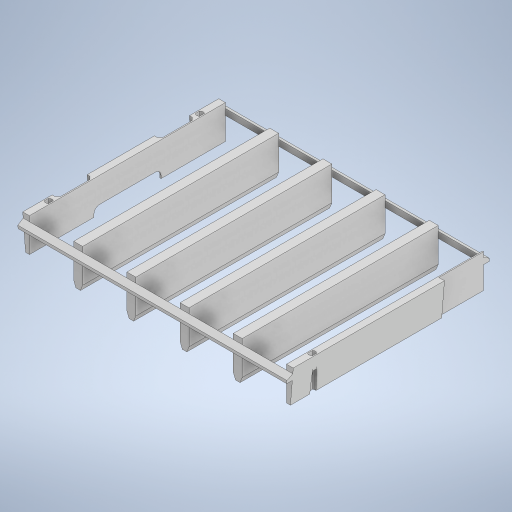
# Autodesk Inventor part: Brackets
Saved by Autodesk Inventor 2023 (Build 270158000, 158)
## iProperties
Created: 2024-03-26
Part Number: Brackets
Material: Generic
Document SubType Name: Modeling
Designer: noname
Density: 1 g/cm^3
Appearance: Default
Author: noname
Autodesk Inventor part; units mm, degrees
ref_plane "YZ Plane" through (0, 0, 0) normal (1, 0, 0) x (0, 1, 0)
ref_plane "XZ Plane" through (0, 0, 0) normal (0, 1, 0) x (-1, 0, 0)
ref_plane "XY Plane" through (0, 0, 0) normal (0, 0, 1) x (1, 0, 0)
sketch "Sketch1" plane through (0, 0, 0) normal (0, 1, 0) x (-1, 0, 0)
  line L0 (0, 0) -> (-96.6, 0) construction
  line L1 (-96.6, 0) -> (-96.6, -70) construction
  line L2 (-96.6, -70) -> (0, -70) construction
  line L3 (0, -70) -> (0, 0) construction
  line L4 (0, 0) -> (-2.4, 0)
  line L5 (-2.4, 0) -> (-2.4, -70)
  line L6 (-2.4, -70) -> (0, -70)
  line L7 (0, -70) -> (0, 0)
  line L8 (-48.3, 0) -> (-48.3, -70)
  line L9 (-96.6, -70) -> (-96.6, 0) construction
  line L10 (-96.6, 0) -> (-94.2, 0)
  line L11 (-94.2, 0) -> (-94.2, -70)
  line L12 (-94.2, -70) -> (-96.6, -70)
  line L13 (-96.6, -70) -> (-96.6, 0)
  line L14 (-18.2, 0) -> (-21.4, 0)
  line L15 (-21.4, 0) -> (-21.4, -70)
  line L16 (-21.4, -70) -> (-18.2, -70)
  line L17 (-18.2, -70) -> (-18.2, 0)
  line L18 (-40.4, 0) -> (-40.4, -70)
  line L19 (-40.4, -70) -> (-37.2, -70)
  line L20 (-37.2, -70) -> (-37.2, 0)
  line L21 (-37.2, 0) -> (-40.4, 0)
  line L22 (-59.4, 0) -> (-59.4, -70)
  line L23 (-59.4, -70) -> (-56.2, -70)
  line L24 (-56.2, -70) -> (-56.2, 0)
  line L25 (-56.2, 0) -> (-59.4, 0)
  line L26 (-78.4, 0) -> (-78.4, -70)
  line L27 (-78.4, -70) -> (-75.2, -70)
  line L28 (-75.2, -70) -> (-75.2, 0)
  line L29 (-75.2, 0) -> (-78.4, 0)
  dimension "d0" = 96.6
  dimension "d1" = 70
  dimension "d2" = 2.4
  dimension "d5" = 19
  dimension "d10" = 19
  dimension "d11" = 3.2
  dimension "d12" = 19
  constraints: 60 end point, 6 parallel, 4 horizontal, 4 symmetric about line, 3 perpendicular, 3 point on line, 2 midpoint, 24 other
  measures "d0" distance between parallel lines of L1 L3
  measures "d1" distance between parallel lines of L0 L2
  measures "d2" distance between parallel lines of L7 L5
  measures "d5" distance of L15.end L18.end
  measures "d10" distance between parallel lines of L5 L15
  measures "d11" distance between parallel lines of L15 L17
  measures "d12" distance between parallel lines of L28 L11
extrude "Extrusion1" add sketch "Sketch1" along normal blind 12
sketch "Sketch2" plane through (0, 0, 0) normal (0, 0, 1) x (1, 0, 0)
  line L0 (18.2, 0) -> (21.4, 0) projected
  line L1 (21.4, 0) -> (21.4, 12) projected
  line L2 (18.2, 12) -> (21.4, 12) projected
  line L3 (18.2, 0) -> (18.2, 12) projected
  line L4 (21.4, 0) -> (18.2, 0) projected
  line L5 (18.2, 0) -> (19, -2)
  line L6 (19, -2) -> (20.6, -2)
  line L7 (20.6, -2) -> (21.4, 0)
  line L8 (18.2, 0) -> (21.4, 0)
  line L9 (37.2, 0) -> (38, -2)
  line L10 (38, -2) -> (39.6, -2)
  line L11 (39.6, -2) -> (40.4, 0)
  line L12 (37.2, 0) -> (40.4, 0)
  line L13 (56.2, 0) -> (57, -2)
  line L14 (57, -2) -> (58.6, -2)
  line L15 (58.6, -2) -> (59.4, 0)
  line L16 (56.2, 0) -> (59.4, 0)
  line L17 (75.2, 0) -> (76, -2)
  line L18 (76, -2) -> (77.6, -2)
  line L19 (77.6, -2) -> (78.4, 0)
  line L20 (75.2, 0) -> (78.4, 0)
  dimension "d17" = 2
  dimension "d18" = 1.6
  dimension "d21" = 19
  constraints: 32 end point, 2 horizontal, 1 equal length, 1 parallel, 24 other
  measures "d17" distance between parallel lines of L0 L6
  measures "d18" distance of L5.end L6.end
  measures "d21" distance of L0.start L9.start
extrude "Extrusion2" add sketch "Sketch2" against normal up to surface (70 mm away) contours L0 L7 L6 L5 | L12 L11 L10 L9 | L16 L15 L14 L13 | L20 L19 L18 L17
sketch "Sketch3" plane through (0, 0, 0) normal (0, 0, 1) x (1, 0, 0)
  line L0 (0, 12) -> (1, 0)
  line L1 (0, 0) -> (0, 12) projected
  line L2 (0, 12) -> (0, 0)
  line L3 (0, 0) -> (1, 0)
  line L4 (40.4, 0) -> (40.4, 12) projected
  line L5 (40.4, 6) -> (56.2, 6) construction
  line L6 (56.2, 0) -> (56.2, 12) projected
  line L7 (48.3, 12) -> (48.3, 0)
  line L8 (96.6, 12) -> (95.6, 0)
  line L9 (96.6, 0) -> (96.6, 12)
  line L10 (96.6, 0) -> (95.6, 0)
  point P0 (48.3, 6)
  dimension "d28" = 1
  constraints: 16 end point, 4 midpoint, 3 symmetric about line, 2 horizontal alignment, 2 vertical, 1 perpendicular
  measures "d28" distance from line of L1 L0.end
extrude "Extrusion3" cut sketch "Sketch3" against normal through all
ref_plane "Work Plane1" through (0, 9, 0) normal (0, 1, 0) x (1, 0, 0)
sketch "Sketch4" plane through (0, 9, 0) normal (0, 1, 0) x (1, 0, 0)
  line L0 (0, 0) -> (2.4, 0) projected
  line L1 (0, 0) -> (96.6, 0)
  line L2 (96.6, 0) -> (96.6, -2)
  line L3 (96.6, -2) -> (0, -2)
  line L4 (0, -2) -> (0, 0)
  line L5 (2.4, 70) -> (0, 70) projected
  line L6 (0, 70) -> (96.6, 70)
  line L7 (96.6, 70) -> (96.6, 72)
  line L8 (96.6, 72) -> (0, 72)
  line L9 (0, 72) -> (0, 70)
  dimension "d32" = 2
  dimension "d36" = 2
  constraints: 16 end point, 4 parallel, 2 horizontal, 2 perpendicular, 2 vertical alignment
  measures "d32" distance between parallel lines of L6 L8
  measures "d36" distance between parallel lines of L3 L1
extrude "Extrusion4" add sketch "Sketch4" against normal blind 1
draft "FaceDraft1" angle 30 pull direction (0, 0, -1) faces at (38.2667, 9, -71.3333) fixed edges at (48.3, 9, -72)
draft "FaceDraft2" angle 30 pull direction (0, 0, 1) faces at (50.9333, 9, 1.3333) fixed edges at (48.3, 9, 2)
sketch "Sketch5" plane through (1, 0, 0) normal (0, 0, 1) x (1, 0, 0)
  line L0 (-0.6667, 8) -> (-0.8462, 10.1547) projected
  line L1 (-1, 10.1547) -> (-0.8462, 10.1547) projected
  line L2 (-1, 10.1547) -> (-1, 8) projected
  line L3 (-0.6667, 8) -> (-1, 8) projected
  line L4 (95.4462, 10.1547) -> (95.2667, 8) projected
  line L5 (95.6, 8) -> (95.2667, 8) projected
  line L6 (95.6, 10.1547) -> (95.6, 8) projected
  line L7 (95.4462, 10.1547) -> (95.6, 10.1547) projected
  point P0 (-1, 0)
extrude "Extrusion5" cut sketch "Sketch5" along normal through all both and the other way through all
sketch "Sketch6" plane through (0, 12, 0) normal (0, 1, 0) x (1, 0, 0)
  line L0 (96.6, 0) -> (96.6, 70) projected
  line L1 (0.3333, 72) -> (96.2667, 72) projected
  line L2 (96.6, 54) -> (94.6, 54)
  line L3 (94.6, 54) -> (94.6, 72)
  line L4 (94.6, 72) -> (96.6, 72)
  line L5 (96.6, 72) -> (96.6, 54)
  line L6 (94.2, 70) -> (94.2, 0) projected
  point P0 (0, 0)
  dimension "d40" = 0.4
  dimension "d41" = 18
  constraints: 8 end point, 2 parallel, 2 point on line, 1 horizontal, 1 perpendicular
  measures "d40" distance between parallel lines of L6 L3
  measures "d41" distance between parallel lines of L1 L2
extrude "Extrusion6" cut sketch "Sketch6" against normal through all
sketch "Sketch7" plane through (0, 12, 0) normal (0, 1, 0) x (1, 0, 0)
  line L0 (0, 70) -> (0, 0) projected
  line L1 (0, 10.5) -> (2, 10.5)
  line L2 (2, 10.5) -> (2, 23)
  line L3 (2, 23) -> (0, 23)
  line L4 (0, 23) -> (0, 10.5)
  line L5 (0, 47) -> (2, 47)
  line L6 (2, 47) -> (2, 59.5)
  line L7 (2, 59.5) -> (0, 59.5)
  line L8 (0, 59.5) -> (0, 47)
  line L9 (2.4, 70) -> (0, 70) projected
  line L10 (0, 0) -> (2.4, 0) projected
  line L11 (2.4, 0) -> (2.4, 70) projected
  point P0 (1.2, 70)
  point P1 (0, 59.5)
  point P2 (0, 23)
  dimension "d45" = 10.5
  dimension "d47" = 10.5
  dimension "d50" = 0.4
  dimension "d63" = 12.5
  dimension "d64" = 12.5
  constraints: 16 end point, 4 parallel, 2 horizontal, 2 perpendicular, 2 point on line, 1 midpoint, 1 vertical alignment
  measures "d45" distance between parallel lines of L7 L9
  measures "d47" distance between parallel lines of L1 L10
  measures "d50" distance between parallel lines of L11 L6
  measures "d63" distance between parallel lines of L5 L7
  measures "d64" distance between parallel lines of L3 L1
extrude "Extrusion7" cut sketch "Sketch7" against normal through all contours L7 L6 L5 L0 | L3 L2 L1 L0
sketch "Sketch8" plane through (0, 0, 0) normal (0, -1, 0) x (1, 0, 0)
  line L0 (2.4, 0) -> (2.4, -70) projected
  line L1 (0, -47) -> (0, -23) projected
  line L2 (2.4, -47.5) -> (0, -47.5)
  line L3 (0, -47.5) -> (0, -22.5)
  line L4 (0, -22.5) -> (2.4, -22.5)
  line L5 (2.4, -22.5) -> (2.4, -47.5)
  line L6 (2, -23) -> (1, -23) projected
  line L7 (0, -23) -> (2, -23) projected
  line L8 (1, -23) -> (0, -23) projected
  line L9 (0, -47) -> (1, -47) projected
  line L10 (1, -47) -> (2, -47) projected
  line L11 (0, -47) -> (1, -47) projected
  line L12 (2, -47) -> (0, -47) projected
  line L13 (2, -47) -> (2, -59.5) projected
  line L14 (2, -59.5) -> (2, -47) projected
  line L15 (2, -10.5) -> (2, -23) projected
  line L16 (2, -23) -> (2, -10.5) projected
  line L17 (2, -23) -> (2.4, -23)
  line L18 (2, -47) -> (2.4, -47)
  point P0 (0, 0)
  point P1 (2.4, -35)
  point P2 (0, -47.5)
  dimension "d53" = 25
  constraints: 12 end point, 5 point on line, 2 midpoint, 2 parallel, 2 perpendicular, 1 horizontal
  measures "d53" distance between parallel lines of L4 L2
extrude "Extrusion8" cut sketch "Sketch8" against normal blind 3 contours L0 L18 L10 L9 L1 L7 L6 L17
fillet "Fillet1" radius 2 2 edges at (2.2, 3, -23) (2.2, 3, -47)
chamfer "Chamfer1" distance 1 angle 45 4 edges at (2, 7.5, -47) (2, 6, -10.5) (2, 6, -59.5) (2, 7.5, -23)
ref_plane "Work Plane2" through (10.3, 12, -70) normal (-1, 0, 0) x (0, 0, 1)
pattern_of_nothing "Rectangular Pattern1"
ref_plane "Work Plane7" through (58.6, -2, -35) normal (0, 0, -1) x (-1, 0, 0)
sketch "Sketch10" plane through (0, 12, 0) normal (0, 1, 0) x (1, 0, 0)
  circle A0 centre (1.3, 8) radius 1.15
  circle A1 centre (1.3, 62) radius 1.15
  line L0 (2.4, 0) -> (2.4, 70) projected
  line L1 (2.4, 35) -> (94.2, 35)
  line L2 (94.2, 70) -> (94.2, 0) projected
  line L3 (40.4, 70) -> (56.2, 70) projected
  line L4 (48.3, 70) -> (48.3, 0)
  line L5 (40.4, 0) -> (56.2, 0) projected
  circle A2 centre (95.3, 8) radius 1.15
  line L6 (0.4, 62.7159) -> (0.4, 7.2841)
  line L7 (2, 7.0876) -> (2, 62.9124)
  line L8 (0, 70) -> (0, 59.5) projected
  line L9 (96.2, 62.7159) -> (96.2, 7.2841)
  line L10 (94.6, 7.0876) -> (94.6, 62.9124)
  point P0 (0, 0)
  point P1 (94.6, 8.9124)
  point P2 (96.2, 7.2841)
  point P3 (96.2, 8.7159)
  point P4 (2, 8.9124)
  point P5 (0.4, 8.7159)
  point P6 (2, 61.0876)
  point P7 (0.4, 61.2841)
  dimension "d74" = 94
  dimension "d75" = 54
  dimension "d76" = 2.3
  dimension "d77" = 0.4
  dimension "d78" = 0.4
  constraints: 12 end point, 5 symmetric about line, 4 midpoint, 4 point on circle, 3 centre point, 2 vertical, 1 vertical alignment, 2 other
  measures "d74" distance of A2.centre A0.centre
  measures "d75" distance of A0.centre A1.centre
  measures "d76" diameter of A0
  measures "d77" distance between parallel lines of L8 L6
  measures "d78" distance between parallel lines of L0 L7
extrude "Extrusion9" cut sketch "Sketch10" against normal through all contours L6 A0 L7 | L6 A1 L7 | A2 L9 L10
ref_plane "Work Plane3" through (29.3, 12, -70) normal (-1, 0, 0) x (0, 0, 1)
ref_plane "Work Plane4" through (48.3, 12, -70) normal (-1, 0, 0) x (0, 0, 1)
ref_plane "Work Plane5" through (67.3, 12, -70) normal (-1, 0, 0) x (0, 0, 1)
ref_plane "Work Plane6" through (86.3, 12, -70) normal (-1, 0, 0) x (0, 0, 1)
body "Solid1"
